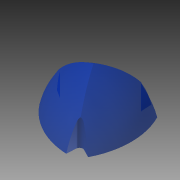
# Autodesk Inventor part: WORK ENVELOPE
Saved by Autodesk Inventor 2013 (Build 170138000, 138)
## iProperties
Created: 2014-01-21
Part Number: WORK ENVELOPE
Material: Generic
Document SubType Name: Modeling
Designer: employee
Density: 1 g/cm^3
Author: employee
Autodesk Inventor part; units mm, degrees
ref_plane "YZ Plane" through (0, 0, 0) normal (1, 0, 0) x (0, 1, 0)
ref_plane "XZ Plane" through (0, 0, 0) normal (0, 1, 0) x (-1, 0, 0)
ref_plane "XY Plane" through (0, 0, 0) normal (0, 0, 1) x (1, 0, 0)
sketch "Sketch1" plane through (0, 0, 0) normal (0, 0, 1) x (1, 0, 0)
  circle A0 centre (0, 0) radius 500
  dimension "d0" = 1000
  constraints: 1 centre point, 1 coincident
  measures "d0" diameter of A0
extrude "Extrusion1" add sketch "Sketch1" along normal blind 1000
sketch "Sketch2" plane through (0, 0, 0) normal (0, 1, 0) x (-1, 0, 0)
  line L0 (144.3376, 0) -> (-72.1688, -125)
  line L1 (-72.1688, -125) -> (-72.1688, 125)
  line L2 (-72.1688, 125) -> (144.3376, 0)
  line L3 (144.3376, 0) -> (144.3376, -72)
  arc A0 (144.3376, 223) -> (144.3376, -367) centre (144.3376, -72) ccw
  line L4 (144.3376, 0) -> (144.3376, 223)
  line L5 (144.3376, -72) -> (144.3376, -367)
  line L6 (144.3376, -367) -> (144.3376, 223)
  line L7 (144.3376, -367) -> (-768.1743, -367)
  line L8 (-768.1743, -367) -> (-768.1743, 1365.1918)
  line L9 (-768.1743, 1365.1918) -> (144.3376, 1365.1918)
  line L10 (144.3376, 1365.1918) -> (144.3376, 223)
  point P0 (0, 0)
  point P1 (0, 0)
  dimension "d4" = 250
  dimension "d5" = 72
  dimension "d6" = 590
  dimension "d7" = 1732.1918
  dimension "d8" = 912.5119
  constraints: 22 end point, 4 collinear, 3 perpendicular, 2 coincident, 2 point on circle, 1 centre point, 1 parallel, 1 tangent, 1 vertical, 7 other
  measures "d4" distance of L0.end L1.end
  measures "d5" distance of L0.start L3.end
  measures "d6" diameter of A0
  measures "d7" distance of L7.end L8.end
  measures "d8" distance of L8.end L9.end
revolve "Revolution1" cut sketch "Sketch2" angle 360 about axis through (-144.3376, 0, 1365.1918) along (0, 0, -1) contours A0 L7 L8 L9 L10
pattern_circular "Circular Pattern1" count 3 over 360 about axis through (0, 0, -10) along (0, 0, 1) of "Revolution1"
sketch "Sketch3" plane through (0, 0, 0) normal (0, 0, -1) x (-1, 0, 0)
  arc A0 (-92.578, -160.3497) -> (185.1559, 0) centre (-72.1688, 125) ccw projected
  arc A1 (185.1559, 0) -> (-92.578, 160.3497) centre (-72.1688, -125) ccw projected
  arc A2 (-92.578, 160.3497) -> (-92.578, -160.3497) centre (144.3376, 0) ccw projected
  circle A3 centre (-72.1688, 125) radius 12.5
  line L0 (-110.2559, 130.4728) -> (-77.8697, 113.8757)
  line L1 (-59.6844, 124.375) -> (-57.8649, 160.7208)
  point P0 (0, 0)
  dimension "d13" = 25
  constraints: 4 end point, 4 point on circle, 2 point on line, 2 tangent, 1 centre point, 1 coincident
  measures "d13" diameter of A3
extrude "Extrusion2" cut sketch "Sketch3" against normal blind 1000 contours A2 A1 L1 A3 L0 | A3
pattern_circular "Circular Pattern2" count 3 over 360 about axis through (0, 0, -10) along (0, 0, 1) of "Extrusion2"
body "Solid1"
